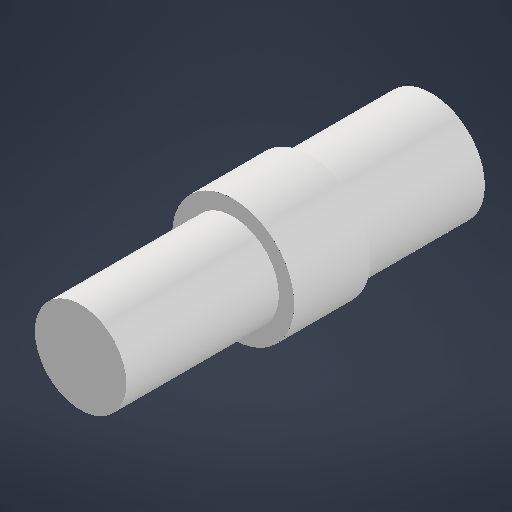
# Autodesk Inventor part: カップリング
Saved by Autodesk Inventor 2026 (Build 300175000, 175)
## iProperties
Created: 2025-10-25
Part Number: カップリング
Material: 一般
Document SubType Name: Modeling
Designer: masak
Density: 1 g/cm^3
Appearance: 既定
Author: masak
Autodesk Inventor part; units mm, degrees
ref_plane "YZ Plane" through (0, 0, 0) normal (1, 0, 0) x (0, 1, 0)
ref_plane "XZ Plane" through (0, 0, 0) normal (0, 1, 0) x (-1, 0, 0)
ref_plane "XY Plane" through (0, 0, 0) normal (0, 0, 1) x (1, 0, 0)
sketch "スケッチ1" plane through (0, 0, 0) normal (0, 0, 1) x (1, 0, 0)
  arc A0 (-2, 1.8875) -> (-2, -1.8875) centre (0, 0) ccw projected
  line L0 (-2, 1.8875) -> (2, 1.8875) projected
  line L1 (2, -1.8875) -> (-2, -1.8875) projected
  arc A1 (2, -1.8875) -> (2, 1.8875) centre (0, 0) ccw projected
  circle A2 centre (0, 0) radius 3.5
  point P0 (0, 0)
  dimension "d0" = 7
  constraints: 1 centre point, 1 coincident
  measures "d0" diameter of A2
extrude "押し出し1" add sketch "スケッチ1" against normal blind 8
sketch "スケッチ2" plane through (0, 0, 0) normal (0, 0, 1) x (1, 0, 0)
  circle A0 centre (0, 0) radius 3.5 projected
  circle A1 centre (0, 0) radius 4
  point P0 (0, 0)
  dimension "d3" = 8
  constraints: 1 centre point, 1 coincident
  measures "d3" diameter of A1
extrude "押し出し2" add sketch "スケッチ2" along normal blind 5 contours A0 | A1
sketch "スケッチ3" plane through (0, 0, 5) normal (0, 0, 1) x (1, 0, 0)
  circle A0 centre (0, 0) radius 3
  dimension "d6" = 6
  constraints: 1 centre point, 1 coincident
  measures "d6" diameter of A0
extrude "押し出し3" add sketch "スケッチ3" along normal blind 10
